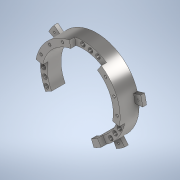
# Autodesk Inventor part: 01
Saved by Autodesk Inventor 2021 (Build 250183000, 183)
## iProperties
Created: 2021-01-14
Part Number: 01
Material: Edelstahl
Document SubType Name: Modeling
Designer: Daniel Dux
Density: 8 g/cm^3
Appearance: Halbpoliert
Mass: 175.616 g
Surface Area: 144.168 cm^2
Volume: 21.952 cm^3
Innenradius: 94,000 mm
Aussenradius: 112,000 mm
m3: 3,500 mm
Stufenhöhe: 7,000 mm
RadiusLoecher: 104,000 mm
m3Kopf: 6,000 mm
MinimalabstandKuehlung: 7,000 mm
InnenradiusOberhalbSchrauben: 98,000 mm
ExtrusionOberhalbSchrauben: 5,000 mm
Plateaudurchmesser: 10,000 mm
Verbindung_d2: 8,000 mm
Plateauhoehe: 18,000 mm
Verbindung_d1: 3,000 mm
Verbindung_d2_tiefe: 15,000 mm
Verbindung_d1_tiefe: 15,000 mm
d85: 98,000 mm
d86: 112,000 mm
d87: 104,000 mm
d88: 5,000 mm
d89: 7,000 mm
d90: 98,000 mm
d91: 5,000 mm
d92: 10,000 mm
ExtrusionHoehenfixierung: 5,000 mm
HoehenfixierungTiefe: 20,000 mm
Author: Daniel Dux
Title: Unterer Mount
Autodesk Inventor part; units mm, degrees
ref_plane "YZ Plane" through (0, 0, 0) normal (1, 0, 0) x (0, 1, 0)
ref_plane "XZ Plane" through (0, 0, 0) normal (0, 1, 0) x (-1, 0, 0)
ref_plane "XY Plane" through (0, 0, 0) normal (0, 0, 1) x (1, 0, 0)
sketch "Skizze2" plane through (0, 0, 0) normal (0, 0, 1) x (1, 0, 0)
  circle A0 centre (0, 0) radius 47
  circle A1 centre (0, 0) radius 56
  circle A2 centre (0, 0) radius 52
  circle A3 centre (0, 52) radius 1.75
  circle A4 centre (-19.8995, 48.0417) radius 1.75
  circle A5 centre (-36.7696, 36.7696) radius 1.75
  circle A6 centre (-48.0417, 19.8995) radius 1.75
  circle A7 centre (-52, 0) radius 1.75
  circle A8 centre (-48.0417, -19.8995) radius 1.75
  circle A9 centre (-36.7696, -36.7696) radius 1.75
  circle A10 centre (-19.8995, -48.0417) radius 1.75
  circle A11 centre (0, -52) radius 1.75
  circle A12 centre (19.8995, -48.0417) radius 1.75
  circle A13 centre (36.7696, -36.7696) radius 1.75
  circle A14 centre (48.0417, -19.8995) radius 1.75
  circle A15 centre (52, 0) radius 1.75
  circle A16 centre (48.0417, 19.8995) radius 1.75
  circle A17 centre (36.7696, 36.7696) radius 1.75
  circle A18 centre (19.8995, 48.0417) radius 1.75
  line L0 (0, 0) -> (0, 56)
  line L1 (0, 0) -> (-10.9251, 54.924)
  line L2 (0, 0) -> (-21.4303, 51.7373)
  line L3 (0, 0) -> (-31.1119, 46.5623)
  line L4 (0, 0) -> (-39.598, 39.598)
  line L5 (0, 0) -> (-46.5623, 31.1119)
  line L6 (0, 0) -> (-51.7373, 21.4303)
  line L7 (0, 0) -> (-54.924, 10.9251)
  line L8 (0, 0) -> (-56, 0)
  line L9 (0, 0) -> (-54.924, -10.9251)
  line L10 (0, 0) -> (-51.7373, -21.4303)
  line L11 (0, 0) -> (-46.5623, -31.1119)
  line L12 (0, 0) -> (-39.598, -39.598)
  line L13 (0, 0) -> (-31.1119, -46.5623)
  line L14 (0, 0) -> (-21.4303, -51.7373)
  line L15 (0, 0) -> (-10.9251, -54.924)
  line L16 (0, 0) -> (0, -56)
  line L17 (0, 0) -> (10.9251, -54.924)
  line L18 (0, 0) -> (21.4303, -51.7373)
  line L19 (0, 0) -> (31.1119, -46.5623)
  line L20 (0, 0) -> (39.598, -39.598)
  line L21 (0, 0) -> (46.5623, -31.1119)
  line L22 (0, 0) -> (51.7373, -21.4303)
  line L23 (0, 0) -> (54.924, -10.9251)
  line L24 (0, 0) -> (56, 0)
  line L25 (0, 0) -> (54.924, 10.9251)
  line L26 (0, 0) -> (51.7373, 21.4303)
  line L27 (0, 0) -> (46.5623, 31.1119)
  line L28 (0, 0) -> (39.598, 39.598)
  line L29 (0, 0) -> (31.1119, 46.5623)
  line L30 (0, 0) -> (21.4303, 51.7373)
  line L31 (0, 0) -> (10.9251, 54.924)
  point P0 (26.1118, 39.0791)
  point P1 (46.0969, -9.1692)
  point P2 (-9.1692, 46.0969)
  point P3 (-46.0969, 9.1692)
  point P4 (9.1692, -46.0969)
  point P5 (-26.1118, -39.0791)
  point P6 (26.1118, -39.0791)
  point P7 (17.9861, -43.4223)
  dimension "d5" = 112
  dimension "d6" = 104
  dimension "d4" = 94
  dimension "d8" = 3.5
  dimension "d11" = 360
  dimension "d15" = 360
  constraints: 64 end point, 17 centre point, 3 coincident, 1 vertical, 1 vertical alignment, 135 other
  measures "d4" diameter of A0
  measures "d8" diameter of A3
extrude "Extrusion2" add sketch "Skizze2" against normal blind 7 contours L24 A15 A2 L23 A0 | A0 L25 A2 A15 L24 | A0 L26 A16 A2 L25 | A0 L27 A2 A16 L26 | L25 A1 L24 A15 A2 | A2 A16 L26 A1 L25 | A2 A15 L24 A1 L23 | A0 L2 A4 A2 L1 | A0 L3 A2 A4 L2 | A0 L4 A5 A2 L3 | A0 L5 A2 A5 L4 | A0 L6 A6 A2 L5 | A0 L7 A2 A6 L6 | A0 L19 A2 A12 L18 | A0 L28 A17 A2 L27 | A0 L29 A2 A17 L28 | A2 A4 L2 A1 L1 | L3 A1 L2 A4 A2 | A2 A5 L4 A1 L3 | L5 A1 L4 A5 A2 | A2 A6 L6 A1 L5 | L7 A1 L6 A6 A2 | A12 A2 L18 | L19 A1 L18 A12 A2 | L27 A1 L26 A16 A2 | A2 A17 L28 A1 L27 | L29 A1 L28 A17 A2 | A12 L18 A2 picked at (19.9797, -47.3914) picked at (20.4216, -48.4382)
sketch "Skizze4" plane through (0, 0, -7) normal (0, 0, -1) x (-1, 0, 0)
  circle A0 centre (0, 0) radius 47
  circle A1 centre (0, 0) radius 56
  circle A2 centre (0, 0) radius 52
  circle A3 centre (0, 52) radius 3
  circle A4 centre (-19.8995, 48.0417) radius 3
  circle A5 centre (-36.7696, 36.7696) radius 3
  circle A6 centre (-48.0417, 19.8995) radius 3
  circle A7 centre (-52, 0) radius 3
  circle A8 centre (-48.0417, -19.8995) radius 3
  circle A9 centre (-36.7696, -36.7696) radius 3
  circle A10 centre (-19.8995, -48.0417) radius 3
  circle A11 centre (0, -52) radius 3
  circle A12 centre (19.8995, -48.0417) radius 3
  circle A13 centre (36.7696, -36.7696) radius 3
  circle A14 centre (48.0417, -19.8995) radius 3
  circle A15 centre (52, 0) radius 3
  circle A16 centre (48.0417, 19.8995) radius 3
  circle A17 centre (36.7696, 36.7696) radius 3
  circle A18 centre (19.8995, 48.0417) radius 3
  circle A19 centre (0, -52) radius 3.5
  circle A20 centre (19.8995, -48.0417) radius 3.5
  line L0 (0, 0) -> (-3.7692, -55.873)
  line L1 (0, 0) -> (24.864, -50.1775)
  line L2 (-54.924, -10.9251) -> (-46.0969, -9.1692) projected
  line L3 (0, 0) -> (-54.924, -10.9251)
  line L4 (46.0969, 9.1692) -> (54.924, 10.9251) projected
  line L5 (0, 0) -> (54.924, 10.9251)
  circle A21 centre (0, 0) radius 49
  line L6 (-26.1118, 39.0791) -> (-31.1119, 46.5623) projected
  line L7 (0, 0) -> (-31.1119, 46.5623)
  line L8 (10.9251, 54.924) -> (9.1692, 46.0969) projected
  line L9 (0, 0) -> (10.9251, 54.924)
  circle A22 centre (0, 52) radius 4
  circle A23 centre (-10.1447, 51.0008) radius 4
  circle A24 centre (-19.8995, 48.0417) radius 4
  circle A25 centre (-28.8897, 43.2364) radius 4
  circle A26 centre (-36.7696, 36.7696) radius 4
  circle A27 centre (-43.2364, 28.8897) radius 4
  circle A28 centre (-48.0417, 19.8995) radius 4
  circle A29 centre (-51.0008, 10.1447) radius 4
  circle A30 centre (-52, 0) radius 4
  circle A31 centre (-51.0008, -10.1447) radius 4
  circle A32 centre (-48.0417, -19.8995) radius 4
  circle A33 centre (-43.2364, -28.8897) radius 4
  circle A34 centre (-36.7696, -36.7696) radius 4
  circle A35 centre (-28.8897, -43.2364) radius 4
  circle A36 centre (-19.8995, -48.0417) radius 4
  circle A37 centre (-10.1447, -51.0008) radius 4
  circle A38 centre (0, -52) radius 4
  circle A39 centre (10.1447, -51.0008) radius 4
  circle A40 centre (19.8995, -48.0417) radius 4
  circle A41 centre (28.8897, -43.2364) radius 4
  circle A42 centre (36.7696, -36.7696) radius 4
  circle A43 centre (43.2364, -28.8897) radius 4
  circle A44 centre (48.0417, -19.8995) radius 4
  circle A45 centre (51.0008, -10.1447) radius 4
  circle A46 centre (52, 0) radius 4
  circle A47 centre (51.0008, 10.1447) radius 4
  circle A48 centre (48.0417, 19.8995) radius 4
  circle A49 centre (43.2364, 28.8897) radius 4
  circle A50 centre (36.7696, 36.7696) radius 4
  circle A51 centre (28.8897, 43.2364) radius 4
  circle A52 centre (19.8995, 48.0417) radius 4
  circle A53 centre (10.1447, 51.0008) radius 4
  circle A54 centre (28.8897, 43.2364) radius 5 construction
  line L10 (0, 0) -> (26.4906, 49.3381)
  arc A55 (54.924, 10.9251) -> (10.9251, 54.924) centre (0, 0) ccw projected
  line L11 (0, 0) -> (35.4449, 43.355)
  line L12 (0, 0) -> (5.5933, 55.72)
  line L13 (0, 0) -> (16.1556, 53.619)
  line L14 (0, 0) -> (-16.1556, 53.619)
  line L15 (0, 0) -> (-5.5933, 55.72)
  line L16 (0, 0) -> (-35.4449, 43.355)
  line L17 (0, 0) -> (-26.4906, 49.3381)
  line L18 (0, 0) -> (-49.3381, 26.4906)
  line L19 (0, 0) -> (-43.355, 35.4449)
  line L20 (0, 0) -> (-55.72, 5.5933)
  line L21 (0, 0) -> (-53.619, 16.1556)
  line L22 (0, 0) -> (-53.619, -16.1556)
  line L23 (0, 0) -> (-55.72, -5.5933)
  line L24 (0, 0) -> (-43.355, -35.4449)
  line L25 (0, 0) -> (-49.3381, -26.4906)
  line L26 (0, 0) -> (-26.4906, -49.3381)
  line L27 (0, 0) -> (-35.4449, -43.355)
  line L28 (0, 0) -> (-5.5933, -55.72)
  line L29 (0, 0) -> (-16.1556, -53.619)
  line L30 (0, 0) -> (16.1556, -53.619)
  line L31 (0, 0) -> (5.5933, -55.72)
  line L32 (0, 0) -> (35.4449, -43.355)
  line L33 (0, 0) -> (26.4906, -49.3381)
  line L34 (0, 0) -> (49.3381, -26.4906)
  line L35 (0, 0) -> (43.355, -35.4449)
  line L36 (0, 0) -> (55.72, -5.5933)
  line L37 (0, 0) -> (53.619, -16.1556)
  line L38 (0, 0) -> (53.619, 16.1556)
  line L39 (0, 0) -> (55.72, 5.5933)
  line L40 (0, 0) -> (43.355, 35.4449)
  line L41 (0, 0) -> (49.3381, 26.4906)
  point P0 (21.756, -43.9053)
  point P1 (-3.2981, -48.8889)
  point P2 (-48.0585, -9.5594)
  point P3 (48.0585, 9.5594)
  point P4 (-46.765, 4.6944)
  point P5 (-45.0017, 13.5592)
  point P6 (-41.4087, 22.2332)
  point P7 (-36.3872, 29.7484)
  point P8 (13.5592, -45.0017)
  point P9 (4.6944, -46.765)
  point P10 (36.3872, 29.7484)
  point P11 (41.4087, 22.2332)
  point P12 (22.2332, 41.4087)
  point P13 (29.7484, 36.3872)
  point P14 (48.4591, 17.4346)
  point P15 (34.652, 38.0984)
  point P16 (17.4346, 48.4591)
  point P17 (-38.0984, 34.652)
  point P18 (-21.9376, 46.5939)
  point P19 (2.437, 51.4423)
  point P20 (-48.4591, 17.4346)
  point P21 (-51.4423, 2.437)
  point P22 (-13.5592, -45.0017)
  point P23 (-22.2332, -41.4087)
  point P24 (41.4087, -22.2332)
  dimension "d19" = 94
  dimension "d21" = 104
  dimension "d20" = 112
  dimension "d22" = 6
  dimension "d25" = 360
  dimension "d27" = 7
  dimension "d28" = 7
  dimension "d29" = 98
  dimension "d33" = 8
  dimension "d36" = 360
  dimension "d38" = 10
  dimension "d41" = 360
  constraints: 76 end point, 53 centre point, 10 coincident, 4 collinear, 4 point on circle, 4 tangent, 1 vertical alignment, 197 other
  measures "d20" diameter of A1
  measures "d22" diameter of A3
  measures "d27" diameter of A19
  measures "d28" diameter of A20
  measures "d29" diameter of A21
  measures "d33" diameter of A22
  measures "d38" diameter of A54
extrude "Extrusion4" add sketch "Skizze4" along normal blind 18 contours A0 L39 A21 A46 L36 | A0 L4 A47 A21 L39 | L36 A21 A45 L37 A0 | A0 L38 A21 A47 L4 | L39 A2 A46 A21 | A21 A47 A2 L39 | L37 A21 A44 L34 A0 | L36 A2 A45 A21 | A21 A46 A2 L36 | A0 L41 A21 A48 L38 | A47 A21 L4 | L4 A21 A47 | L2 A31 A21 L23 A0 | A0 L22 A21 A31 L2 | L6 A25 A21 L17 A0 | A0 L16 A21 A25 L6 | L8 A53 A21 L13 A0 | A0 L12 A21 A53 L8 | L10 A21 A51 L11 A0 | A0 L13 A21 A52 L10 | L11 A21 A50 L40 A0 | A0 L15 A21 A22 L12 | L14 A21 A23 L15 A0 | A0 L17 A21 A24 L14 | A0 L19 A21 A26 L16 | L18 A21 A27 L19 A0 | A0 L21 A21 A28 L18 | L20 A21 A29 L21 A0 | A0 L23 A21 A30 L20 | A0 L25 A21 A32 L22 | L24 A21 A33 L25 A0 | A0 L27 A21 A34 L24 | L26 A21 A35 L27 A0 | L40 A21 A49 L41 A0 | A46 A2 A15 A21 | A21 A46 | A21 L4 A2 A47 | L39 A1 A46 A2 | A2 A47 A1 L39 | L37 A2 A44 A21 | A21 A45 A2 L37 | A45 A2 A21 | A21 A45 | A21 A15 A2 A46 | L36 A1 A45 A2 | A2 A46 A1 L36 | L38 A2 A47 A21 | A21 A48 A2 L38 | A21 A47 A2 L4 | A31 A21 L2 | L2 A21 A31 | A25 A21 L6 | L6 A21 A25 | A53 A21 L8 | L8 A21 A53 | L10 A2 A51 A21 | A21 A52 A2 L10 | L11 A2 A50 A21 | A21 A51 A2 L11 | L12 A2 A53 A21 | A21 A22 A2 L12 | L13 A2 A52 A21 | A21 A53 A2 L13 | L14 A2 A23 A21 | A21 A24 A2 L14 | L15 A2 A22 A21 | A21 A23 A2 L15 | L16 A2 A25 A21 | A21 A26 A2 L16 | L17 A2 A24 A21 | A21 A25 A2 L17 | L18 A2 A27 A21 | A21 A28 A2 L18 | L19 A2 A26 A21 | A21 A27 A2 L19 | L20 A2 A29 A21 | A21 A30 A2 L20 | L21 A2 A28 A21 | A21 A29 A2 L21 | L22 A2 A31 A21 | A21 A32 A2 L22 | L23 A2 A30 A21 | A21 A31 A2 L23 | L24 A2 A33 A21 | A21 A34 A2 L24 | L25 A2 A32 A21 | A21 A33 A2 L25 | L26 A2 A35 A21 | L27 A2 A34 A21 | A21 A35 A2 L27 | A21 A44 A2 L34 | L40 A2 A49 A21 | A21 A50 A2 L40 | L41 A2 A48 A21 | A21 A49 A2 L41 | A46 A2 A15 | A2 L4 A47 | A44 A2 A14 A21 | A21 A44 | L37 A1 A44 A2 | A2 A45 A1 L37 | A45 A2 | A48 A21 | A21 A16 A2 A48 | L38 A1 A47 A2 | A2 A48 A1 L38 | A2 A47 L4 | A21 A31 A2 L2 | L2 A2 A31 A21 | L6 A2 A25 A21 | A21 A25 A2 L6 | L8 A2 A53 A21 | A21 A53 A2 L8 | A51 A2 A21 | A21 A51 | A52 A21 | A21 A18 A2 A52 | L10 A1 A51 A2 | A2 A52 A1 L10 | A50 A2 A17 A21 | A21 A50 | L11 A1 A50 A2 | A2 A51 A1 L11 | A22 A21 | A21 A3 A2 A22 | L12 A1 A53 A2 | A2 A22 A1 L12 | A52 A2 A18 A21 | L13 A1 A52 A2 | A2 A53 A1 L13 | A23 A2 A21 | A21 A23 | A24 A21 | A21 A4 A2 A24 | L14 A1 A23 A2 | A2 A24 A1 L14 | A22 A2 A3 A21 | L15 A1 A22 A2 | A2 A23 A1 L15 | A26 A21 | A21 A5 A2 A26 | L16 A1 A25 A2 | A2 A26 A1 L16 | A24 A2 A4 A21 | L17 A1 A24 A2 | A2 A25 A1 L17 | A27 A2 A21 | A21 A27 | A28 A21 | A21 A6 A2 A28 | L18 A1 A27 A2 | A2 A28 A1 L18 | A26 A2 A5 A21 | L19 A1 A26 A2 | A2 A27 A1 L19 | A29 A2 A21 | A21 A29 | A30 A21 | A21 A7 A2 A30 | L20 A1 A29 A2 | A2 A30 A1 L20 | A28 A2 A6 A21 | L21 A1 A28 A2 | A2 A29 A1 L21 | A32 A21 | A21 A8 A2 A32 | L22 A1 A31 A2 | A2 A32 A1 L22 | A30 A2 A7 A21 | L23 A1 A30 A2 | A2 A31 A1 L23 | A33 A2 A21 | A21 A33 | A34 A21 | A21 A9 A2 A34 | L24 A1 A33 A2 | A2 A34 A1 L24 | A32 A2 A8 A21 | L25 A1 A32 A2 | A2 A33 A1 L25 | A35 A2 A21 | A21 A35 | L26 A1 A35 A2 | A34 A2 A9 A21 | L27 A1 A34 A2 | A2 A35 A1 L27 | A21 A14 A2 A44 | A2 A44 A1 L34 | A49 A2 A21 | A21 A49 | A21 A17 A2 A50 | L40 A1 A49 A2 | A2 A50 A1 L40 | A48 A2 A16 A21 | L41 A1 A48 A2 | A2 A49 A1 L41 | A44 A2 A14 | A2 A16 A48 | L2 A31 A2 | A2 A31 L2 | L6 A25 A2 | A2 A25 L6 | L8 A53 A2 | A2 A53 L8 | A51 A2 | A2 A18 A52 | A50 A2 A17 | A2 A3 A22 | A23 A2 | A2 A4 A24 | A2 A5 A26 | A27 A2 | A2 A6 A28 | A29 A2 | A2 A7 A30 | A2 A8 A32 | A33 A2 | A2 A9 A34 | A35 A2 | A49 A2
sketch "Skizze5" plane through (0, 0, -25) normal (0, 0, -1) x (-1, 0, 0)
  circle A0 centre (0, 0) radius 51.5
  point P0 (0, 51.5)
  point P1 (-10.0472, 50.5104)
  point P2 (-19.7082, 47.5798)
  point P3 (-28.6119, 42.8207)
  point P4 (-36.416, 36.416)
  point P5 (-42.8207, 28.6119)
  point P6 (-47.5798, 19.7082)
  point P7 (-50.5104, 10.0472)
  point P8 (-51.5, 0)
  point P9 (-50.5104, -10.0472)
  point P10 (-47.5798, -19.7082)
  point P11 (-42.8207, -28.6119)
  point P12 (-36.416, -36.416)
  point P13 (-28.6119, -42.8207)
  point P14 (-19.7082, -47.5798)
  point P15 (-10.0472, -50.5104)
  point P16 (0, -51.5)
  point P17 (10.0472, -50.5104)
  point P18 (19.7082, -47.5798)
  point P19 (28.6119, -42.8207)
  point P20 (36.416, -36.416)
  point P21 (42.8207, -28.6119)
  point P22 (47.5798, -19.7082)
  point P23 (50.5104, -10.0472)
  point P24 (51.5, 0)
  point P25 (50.5104, 10.0472)
  point P26 (47.5798, 19.7082)
  point P27 (42.8207, 28.6119)
  point P28 (36.416, 36.416)
  point P29 (28.6119, 42.8207)
  point P30 (19.7082, 47.5798)
  point P31 (10.0472, 50.5104)
  dimension "d45" = 103
  dimension "d48" = 360
  constraints: 1 coincident, 1 vertical alignment, 35 other
hole "Bohrung2" at (-28.6119, 42.8207, -25) at (-42.8207, 28.6119, -25) at (-10.0472, -50.5104, -25) at (50.5104, 10.0472, -25) at (42.8207, 28.6119, -25) at (28.6119, -42.8207, -25) at (-50.5104, 10.0472, -25) direction (0, 0, 1) diameter 8 depth 15
sketch "Skizze7" plane through (0, 0, -25) normal (0, 0, -1) x (-1, 0, 0)
  circle A0 centre (0, 0) radius 49
  circle A1 centre (0, 0) radius 56
  circle A2 centre (0, 0) radius 52
  circle A3 centre (0, 52) radius 2.5
  circle A4 centre (-19.8995, 48.0417) radius 2.5
  circle A5 centre (-36.7696, 36.7696) radius 2.5
  circle A6 centre (-48.0417, 19.8995) radius 2.5
  circle A7 centre (-52, 0) radius 2.5
  circle A8 centre (-48.0417, -19.8995) radius 2.5
  circle A9 centre (-36.7696, -36.7696) radius 2.5
  circle A10 centre (-19.8995, -48.0417) radius 2.5
  circle A11 centre (0, -52) radius 2.5
  circle A12 centre (19.8995, -48.0417) radius 2.5
  circle A13 centre (36.7696, -36.7696) radius 2.5
  circle A14 centre (48.0417, -19.8995) radius 2.5
  circle A15 centre (52, 0) radius 2.5
  circle A16 centre (48.0417, 19.8995) radius 2.5
  circle A17 centre (36.7696, 36.7696) radius 2.5
  circle A18 centre (19.8995, 48.0417) radius 2.5
  circle A19 centre (0, -52) radius 3.5
  circle A20 centre (19.8995, -48.0417) radius 3.5
  line L0 (0, 0) -> (-3.7692, -55.873)
  line L1 (0, 0) -> (24.864, -50.1775)
  line L2 (-54.924, -10.9251) -> (-48.0585, -9.5594)
  line L3 (0, 0) -> (-54.924, -10.9251)
  line L4 (48.0585, 9.5594) -> (54.924, 10.9251)
  line L5 (0, 0) -> (54.924, 10.9251)
  circle A21 centre (0, 0) radius 49
  line L6 (-27.2229, 40.742) -> (-31.1119, 46.5623)
  line L7 (0, 0) -> (-31.1119, 46.5623)
  line L8 (10.9251, 54.924) -> (9.5594, 48.0585)
  line L9 (0, 0) -> (10.9251, 54.924)
  circle A22 centre (0, 52) radius 2.5
  circle A23 centre (-10.1447, 51.0008) radius 2.5
  circle A24 centre (-19.8995, 48.0417) radius 2.5
  circle A25 centre (-28.8897, 43.2364) radius 2.5
  circle A26 centre (-36.7696, 36.7696) radius 2.5
  circle A27 centre (-43.2364, 28.8897) radius 2.5
  circle A28 centre (-48.0417, 19.8995) radius 2.5
  circle A29 centre (-51.0008, 10.1447) radius 2.5
  circle A30 centre (-52, 0) radius 2.5
  circle A31 centre (-51.0008, -10.1447) radius 2.5
  circle A32 centre (-48.0417, -19.8995) radius 2.5
  circle A33 centre (-43.2364, -28.8897) radius 2.5
  circle A34 centre (-36.7696, -36.7696) radius 2.5
  circle A35 centre (-28.8897, -43.2364) radius 2.5
  circle A36 centre (-19.8995, -48.0417) radius 2.5
  circle A37 centre (-10.1447, -51.0008) radius 2.5
  circle A38 centre (0, -52) radius 2.5
  circle A39 centre (10.1447, -51.0008) radius 2.5
  circle A40 centre (19.8995, -48.0417) radius 2.5
  circle A41 centre (28.8897, -43.2364) radius 2.5
  circle A42 centre (36.7696, -36.7696) radius 2.5
  circle A43 centre (43.2364, -28.8897) radius 2.5
  circle A44 centre (48.0417, -19.8995) radius 2.5
  circle A45 centre (51.0008, -10.1447) radius 2.5
  circle A46 centre (52, 0) radius 2.5
  circle A47 centre (51.0008, 10.1447) radius 2.5
  circle A48 centre (48.0417, 19.8995) radius 2.5
  circle A49 centre (43.2364, 28.8897) radius 2.5
  circle A50 centre (36.7696, 36.7696) radius 2.5
  circle A51 centre (28.8897, 43.2364) radius 2.5
  circle A52 centre (19.8995, 48.0417) radius 2.5
  circle A53 centre (10.1447, 51.0008) radius 2.5
  circle A54 centre (28.8897, 43.2364) radius 5 construction
  line L10 (0, 0) -> (26.4906, 49.3381)
  arc A55 (54.924, 10.9251) -> (10.9251, 54.924) centre (0, 0) ccw
  line L11 (0, 0) -> (35.4449, 43.355)
  line L12 (0, 0) -> (5.5933, 55.72)
  line L13 (0, 0) -> (16.1556, 53.619)
  line L14 (0, 0) -> (-16.1556, 53.619)
  line L15 (0, 0) -> (-5.5933, 55.72)
  line L16 (0, 0) -> (-35.4449, 43.355)
  line L17 (0, 0) -> (-26.4906, 49.3381)
  line L18 (0, 0) -> (-49.3381, 26.4906)
  line L19 (0, 0) -> (-43.355, 35.4449)
  line L20 (0, 0) -> (-55.72, 5.5933)
  line L21 (0, 0) -> (-53.619, 16.1556)
  line L22 (0, 0) -> (-53.619, -16.1556)
  line L23 (0, 0) -> (-55.72, -5.5933)
  line L24 (0, 0) -> (-43.355, -35.4449)
  line L25 (0, 0) -> (-49.3381, -26.4906)
  line L26 (0, 0) -> (-26.4906, -49.3381)
  line L27 (0, 0) -> (-35.4449, -43.355)
  line L28 (0, 0) -> (-5.5933, -55.72)
  line L29 (0, 0) -> (-16.1556, -53.619)
  line L30 (0, 0) -> (16.1556, -53.619)
  line L31 (0, 0) -> (5.5933, -55.72)
  line L32 (0, 0) -> (35.4449, -43.355)
  line L33 (0, 0) -> (26.4906, -49.3381)
  line L34 (0, 0) -> (49.3381, -26.4906)
  line L35 (0, 0) -> (43.355, -35.4449)
  line L36 (0, 0) -> (55.72, -5.5933)
  line L37 (0, 0) -> (53.619, -16.1556)
  line L38 (0, 0) -> (53.619, 16.1556)
  line L39 (0, 0) -> (55.72, 5.5933)
  line L40 (0, 0) -> (43.355, 35.4449)
  line L41 (0, 0) -> (49.3381, 26.4906)
  circle A56 centre (0, 0) radius 66
  line L42 (0, 0) -> (51.097, 41.7744)
  line L43 (0, 0) -> (58.1485, 31.2211)
  line L44 (0, 0) -> (6.5921, -65.67)
  line L45 (0, 0) -> (19.0405, -63.1938)
  line L46 (0, 0) -> (-63.1938, 19.0405)
  line L47 (0, 0) -> (-65.67, 6.5921)
  circle A57 centre (0, 0) radius 61
  line L48 (0, 0) -> (-59.8279, 11.9005)
  line L49 (0, 0) -> (50.7196, 33.8898)
  line L50 (0, 0) -> (11.9005, -59.8279)
  line L51 (0, 0) -> (-41.7744, -51.097)
  line L52 (0, 0) -> (-31.2211, -58.1485)
  line L53 (0, 0) -> (-33.8898, -50.7196)
  line L54 (-31.1119, -46.5623) -> (-26.1118, -39.0791) projected
  line L55 (52, 0) -> (48.0417, -19.8995)
  line L56 (0, 0) -> (51.0008, -10.1447)
  line L57 (0, 52) -> (-19.8995, 48.0417)
  line L58 (0, 0) -> (-10.1447, 51.0008)
  circle A58 centre (-48.0417, -19.8995) radius 3 projected
  line L59 (-48.0417, -19.8995) -> (-36.7696, -36.7696)
  line L60 (0, 0) -> (-43.2364, -28.8897)
  point P0 (21.756, -43.9053)
  point P1 (-3.2981, -48.8889)
  point P2 (-48.755, 4.8941)
  point P3 (-46.9166, 14.1361)
  point P4 (-43.1708, 23.1793)
  point P5 (-37.9356, 31.0143)
  point P6 (14.1361, -46.9166)
  point P7 (4.8941, -48.755)
  point P8 (37.9356, 31.0143)
  point P9 (43.1708, 23.1793)
  point P10 (23.1793, 43.1708)
  point P11 (31.0143, 37.9356)
  point P12 (45.2701, 18.7515)
  point P13 (34.6482, 34.6482)
  point P14 (18.7515, 45.2701)
  point P15 (-34.6482, 34.6482)
  point P16 (-18.7515, 45.2701)
  point P17 (0, 49)
  point P18 (-45.2701, 18.7515)
  point P19 (-49, 0)
  point P20 (50.0209, -9.9498)
  point P21 (-9.9498, 50.0209)
  point P22 (-42.4056, -28.3345)
  dimension "d74" = 112
  dimension "d93" = 132
  dimension "d73" = 98
  dimension "d75" = 104
  dimension "d76" = 5
  dimension "d77" = 360
  dimension "d78" = 7
  dimension "d79" = 7
  dimension "d80" = 98
  dimension "d81" = 5
  dimension "d82" = 360
  dimension "d83" = 10
  dimension "d84" = 360
  dimension "d96" = 122
  constraints: 120 end point, 56 centre point, 14 collinear, 12 coincident, 10 point on circle, 7 point on line, 4 tangent, 3 midpoint, 1 perpendicular, 207 other
  measures "d73" diameter of A0
  measures "d75" diameter of A2
  measures "d76" diameter of A3
  measures "d78" diameter of A19
  measures "d79" diameter of A20
  measures "d80" diameter of A21
  measures "d81" diameter of A22
  measures "d83" diameter of A54
  measures "d96" diameter of A57
extrude "Extrusion5" add sketch "Skizze7" against normal blind 5 contours L47 A57 L48 A1 | A1 L48 A57 L46 | L52 A57 L53 A1 | A1 L53 A57 L51 | L42 A57 L49 A1 | A1 L49 A57 L43 | L47 A56 L46 A57 | L52 A56 L51 A57 | L42 A56 L43 A57
hole "Bohrung3" at (-50.7196, 33.8898, -25) at (-11.9005, -59.8279, -25) at (59.8279, 11.9005, -25) at (33.8898, -50.7196, -25) direction (0, 0, 1) diameter 2.5 end through all
hole "Bohrung4" at (-50.0209, -9.9498, -25) at (9.9498, 50.0209, -25) at (42.4056, -28.3345, -25) direction (0, 0, 1) diameter 6 end through all
equation "\"d5\" = Aussenradius"
equation "\"d6\" = RadiusLoecher"
equation "\"d4\" = Innenradius"
equation "\"d8\" = m3"
equation "\"d17\" = Stufenhöhe"
equation "\"d19\" = Innenradius"
equation "\"d21\" = RadiusLoecher"
equation "\"d20\" = Aussenradius"
equation "\"d22\" = m3Kopf"
equation "\"d27\" = MinimalabstandKuehlung"
equation "\"d28\" = MinimalabstandKuehlung"
equation "\"d29\" = InnenradiusOberhalbSchrauben"
equation "\"Innenradius\" = 94"
equation "\"Aussenradius\" = 112"
equation "\"m3\" = 3.5"
equation "\"Stufenhöhe\" = 7"
equation "\"RadiusLoecher\" = 104"
equation "\"m3Kopf\" = 6"
equation "\"MinimalabstandKuehlung\" = 7"
equation "\"InnenradiusOberhalbSchrauben\" = 98"
equation "\"ExtrusionOberhalbSchrauben\" = 5"
equation "\"Plateaudurchmesser\" = 10"
equation "\"Verbindung_d2\" = 8"
equation "\"Plateauhoehe\" = 18"
equation "\"Verbindung_d1\" = 3"
equation "\"Verbindung_d2_tiefe\" = 15"
equation "\"Verbindung_d1_tiefe\" = 15"
equation "\"ExtrusionHoehenfixierung\" = 5"
equation "\"HoehenfixierungTiefe\" = 20"
equation "\"d85\" = 98"
equation "\"d86\" = 112"
equation "\"d87\" = 104"
equation "\"d88\" = 5"
equation "\"d89\" = 7"
equation "\"d90\" = 98"
equation "\"d91\" = 5"
equation "\"d92\" = 10"
equation "\"HoehenfixierungGewinde\" = 2.5"
